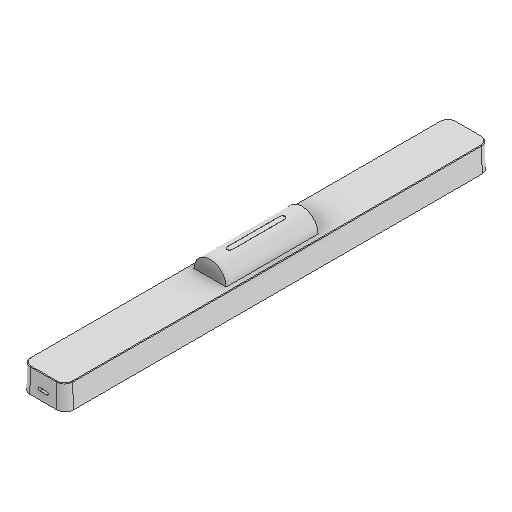
# Autodesk Inventor part: 燈
Saved by Autodesk Inventor 2025.2 (Build 292293000, 293)
## iProperties
Created: 2025-06-18
Part Number: 燈
Material: 一般
Document SubType Name: Modeling
Designer: jna1j
Density: 1 g/cm^3
Appearance: 預設
Author: jna1j
Autodesk Inventor part; units mm, degrees
ref_plane "YZ Plane" through (0, 0, 0) normal (1, 0, 0) x (0, 1, 0)
ref_plane "XZ Plane" through (0, 0, 0) normal (0, 1, 0) x (-1, 0, 0)
sketch "草圖1" plane through (0, 0, 0) normal (0, 0, 1) x (1, 0, 0)
  line L0 (-17.8, 0) -> (17.8, 0)
  line L1 (-17.8, 0) -> (17.8, 0) construction
  line L2 (-18.5, -20.4831) -> (18.5, -20.4831)
  line L3 (-17.8, 0) -> (-18.5, -20.4831)
  line L4 (17.8, 0) -> (18.5, -20.4831)
  arc A0 (17.8, 0) -> (-17.8, 0) centre (0, -499.6831) ccw
  circle A1 centre (0, 0) radius 13.6791
  line L5 (0, 13.6791) -> (0, -20.4831) construction
  line L6 (-2.1, 13.5169) -> (2.1, 13.5169)
  point P0 (0, 0)
  point P1 (0, 0)
  point P2 (-13.6785, 0.1298)
  point P3 (13.6785, 0.1298)
  point P4 (0, 0.3169)
  point P5 (0, 13.5169)
  dimension "d0" = 35.6
  dimension "d2" = 37
  dimension "d15" = 500
  dimension "d32" = 20.8
  dimension "d34" = 34
  dimension "d35" = 4.2
  constraints: 14 end point, 5 point on circle, 4 horizontal, 4 midpoint, 2 centre point, 2 coincident, 2 vertical alignment, 1 collinear, 1 vertical
  measures "d0" distance of L0.start L0.end
  measures "d2" distance of L2.start L2.end
  measures "d15" radius of A0
  measures "d32" distance from line of L2 point (0, 0.317)
  measures "d34" distance between parallel lines of L2 L6
  measures "d35" distance of L6.start L6.end
extrude "擠出1" add sketch "草圖1" along normal mid plane 360 contours A1 A0 L0 | A1 L0 | L0 A1 A0 | L0 L4 L2 L3 A1 | L0 A0 A1
extrude "擠出4" add sketch "草圖1" along normal mid plane 77.8 contours A0 A1 L6 | L6 A1
fillet "圓角3" radius 7 4 edges at (-18.15, -10.2415, -180) (18.15, -10.2415, -180) (18.15, -10.2415, 180) (-18.15, -10.2415, 180)
fillet "圓角4" radius 0.5 8 edges at (16.1323, 0.0566, 177.5316) (0, 0.3169, 180) (-16.1323, 0.0566, 177.5316) (-17.8, 0, 0) (-16.1323, 0.0566, -177.5316) (0, 0.3169, -180) (16.1338, 0.0566, -177.5299) (17.8, 0, 0)
sketch "草圖4" plane through (0, 0, 180) normal (0, 0, 1) x (1, 0, 0)
  line L0 (-2.94, -11.2431) -> (2.94, -11.2431)
  line L1 (2.94, -11.2431) -> (2.94, -13.6831)
  line L2 (2.94, -13.6831) -> (-2.94, -13.6831)
  line L3 (-2.94, -13.6831) -> (-2.94, -11.2431)
  circle A0 centre (2.94, -12.4631) radius 1.22
  circle A1 centre (-2.94, -12.4631) radius 1.22
  line L4 (-4.16, -12.4631) -> (4.16, -12.4631) construction
  arc A2 (10.8062, -0.3) -> (-10.8062, -0.3) centre (0, -499.6831) ccw projected
  line L5 (-11.4959, -20.4831) -> (11.4959, -20.4831) projected
  point P0 (0, 0)
  point P1 (0, -12.4631)
  point P2 (0, -0.1831)
  dimension "d28" = 2.44
  dimension "d30" = 8.32
  dimension "d31" = 6.8
  constraints: 10 end point, 5 point on circle, 3 midpoint, 2 centre point, 2 parallel, 1 horizontal, 1 horizontal alignment, 1 perpendicular, 1 vertical alignment
  measures "d28" distance of L2.end L0.start
  measures "d30" distance of L4.start L4.end
  measures "d31" distance between parallel lines of L5 L2
ref_plane "工作平面4" through (0, 13.6791, 0) normal (0, -1, 0) x (1, 0, 0)
sketch "草圖5" plane through (0, 13.6791, 0) normal (0, -1, 0) x (1, 0, 0)
  line L0 (0, 22.28) -> (0, -22.28) construction
  line L1 (2.1, 22.28) -> (2.1, -22.28)
  line L2 (-2.1, -22.28) -> (-2.1, 22.28)
  arc A0 (2.1, 22.28) -> (-2.1, 22.28) centre (0, 22.28) ccw
  arc A1 (-2.1, -22.28) -> (2.1, -22.28) centre (0, -22.28) ccw
  line L3 (0, 24.38) -> (0, -24.38) construction
  point P0 (0, 0)
  point P1 (0, 0)
  point P2 (0, 0)
  dimension "d36" = 4.2
  dimension "d37" = 48.76
  constraints: 10 end point, 6 point on circle, 4 tangent, 2 centre point, 2 midpoint, 1 coincident, 1 parallel, 1 vertical
  measures "d36" distance between parallel lines of L1 L2
  measures "d37" distance of L3.start L3.end
extrude "擠出6" cut sketch "草圖5" along normal blind 0.3
extrude "擠出7" cut sketch "草圖4" against normal blind 6.8
